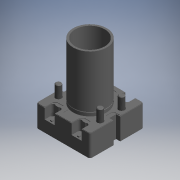
# Autodesk Inventor part: SLZ_63_Abdeckkappe#
Saved by Autodesk Inventor 2017.3 (Build 213256000, 256)
## iProperties
Part Number: SLZ_63_Abdeckkappe#
Material: Generic
Catalog Web Link: www.cadenas.de
Description: AbdeckKappe_SLZ63-Control-Tec
Vendor: ROSEKRIEGER
Document SubType Name: Modeling
Designer: partserver
Manufacturer: ROSEKRIEGER
Mass: 177.566 g
Surface Area: 701.344 cm^2
Volume: 177.566 cm^3
Density: 1 g/cm^3
Appearance: PSOLRGB-128-128-128
Category: PARTsolutions
Company: ROSEKRIEGER
Title: SLZ_63_Abdeckkappe#
Author: Cadenas PARTsolutions
Comments: Control-Tec
PSOL_IDENT_0: {$CADENAS_DATA\23d-libs\rose_krieger\linearkomponenten\pool_lineartechnik\_hubsaeule_zyliinder\elekt
PSOL_IDENT_1: rozylinder\elekzyl_slz63\parts\slz63_plfl_abdeck_kappe.prj},189 {VTYP=3D},{NB=SLZ_63_Abdeckkappe#},{
PSOL_IDENT_2: LINA=SLZ_63_Abdeckkappe#},{NN=AbdeckKappe_SLZ63},{DATE=02.12.2020 11:16:21},{GEOMDATE=06.03.2017 15:
PSOL_IDENT_3: 22:00},{VERSION=},{LINEID=10},{WBVAR=},{WBNUMERIC=}  {NB=SLZ_63_Abdeckkappe#},{LINA=SLZ_63_Abdeckkap
PSOL_IDENT_4: pe#},{KT=DUMMY},{IDNR=},{CODE=TQ3},{ARTIKEL=Elektrozylinder },{TYPE=SLZ 63 KG P PL},{BEST=SLZ_63_Abd
PSOL_IDENT_5: eckkappe},{VARIANTE=PL},{SPINDEL=KG 25x10},{SPINDELCODE=3.000},{SCHUTZARTVIS=IP54},{SCHUTZART=1},{HU
PSOL_IDENT_6: B1=0,[0:100]},{HINWEINBAUX=Hub + 288,5 mm},{DUMMYDURCH=10.000},{DUMMYLAENG=20.000},{HILFEHUB=105},{L
PSOL_IDENT_7: AENDOPPROFIL=184.500},{RF=1.000},{GRUNDKOE=288.500},{A=100},{B=80},{C=100},{D=125},{E=238},{F=40},{G=
PSOL_IDENT_8: M16x1.5},{H=104},{K=125},{L=105},{M=48},{N=56.5},{O=86},{P=18.5},{PPATH=sbl_lz70p_plfl.prj}
NB: SLZ_63_Abdeckkappe#
NN: AbdeckKappe_SLZ63
NT: Control-Tec
NBSYN: $BEST.#
LINA: SLZ_63_Abdeckkappe#
CATALOG: RK Rose+Krieger
ARTIKEL: Elektrozylinder
TYPE: SLZ 63 KG P PL
BEST: SLZ_63_Abdeckkappe
VARIANTE: PL
SPINDEL: KG 25x10
SPINDELCODE: 3
SCHUTZARTVIS: IP54
SCHUTZART: 1
HUB1: 0,[0:100]
HINWEINBAUX: Hub + 288,5 mm
DUMMYDURCH: 10
DUMMYLAENG: 20
HILFEHUB: 105
LAENDOPPROFIL: 184.5
RF: 1
GRUNDKOE: 288.5
A: 100
B: 80
C: 100
D: 125
E: 238
F: 40
G: M16x1.5
H: 104
K: 125
L: 105
M: 48
N: 56.5
O: 86
P: 18.5
SUPPLIER: ROSEKRIEGER
ARTICLENO: SLZ_63_Abdeckkappe#
BOMINFO: SLZ_63_Abdeckkappe#
CREATOR: CADENAS GmbH
Autodesk Inventor part; units mm, degrees
sketch "Sketch_2" plane through (0, 0, 0) normal (0, 0, 1) x (1, 0, 0)
  arc A0 (-40, -37) -> (-37, -40) centre (-37, -37) ccw
  line L0 (-37, -40) -> (37, -40)
  arc A1 (37, -40) -> (40, -37) centre (37, -37) ccw
  line L1 (40, -37) -> (40, -5)
  line L2 (40, -5) -> (33.9, -5)
  line L3 (33.9, -5) -> (33.9, 5)
  line L4 (33.9, 5) -> (40, 5)
  line L5 (40, 5) -> (40, 37)
  arc A2 (40, 37) -> (37, 40) centre (37, 37) ccw
  line L6 (37, 40) -> (-37, 40)
  arc A3 (-37, 40) -> (-40, 37) centre (-37, 37) ccw
  line L7 (-40, 37) -> (-40, 5)
  line L8 (-40, 5) -> (-33.9, 5)
  line L9 (-33.9, 5) -> (-33.9, -5)
  line L10 (-33.9, -5) -> (-40, -5)
  line L11 (-40, -5) -> (-40, -37)
  circle A4 centre (31, 16) radius 4.5
  circle A5 centre (31, -16) radius 4.5
  circle A6 centre (-31, 16) radius 4.5
  circle A7 centre (-31, -16) radius 4.5
  constraints: 24 end point, 8 centre point, 8 point on circle
extrude "Extrusion1" add sketch "Sketch_2" along normal blind 22
sketch "Sketch_1" plane through (0, 0, 22) normal (0, 0, 1) x (1, 0, 0)
  arc A0 (-40, -37) -> (-37, -40) centre (-37, -37) ccw
  line L0 (-37, -40) -> (37, -40)
  arc A1 (37, -40) -> (40, -37) centre (37, -37) ccw
  line L1 (40, -37) -> (40, -5)
  line L2 (40, -5) -> (33.9, -5)
  line L3 (33.9, -5) -> (33.9, 5)
  line L4 (33.9, 5) -> (40, 5)
  line L5 (40, 5) -> (40, 37)
  arc A2 (40, 37) -> (37, 40) centre (37, 37) ccw
  line L6 (37, 40) -> (-37, 40)
  arc A3 (-37, 40) -> (-40, 37) centre (-37, 37) ccw
  line L7 (-40, 37) -> (-40, 5)
  line L8 (-40, 5) -> (-33.9, 5)
  line L9 (-33.9, 5) -> (-33.9, -5)
  line L10 (-33.9, -5) -> (-40, -5)
  line L11 (-40, -5) -> (-40, -37)
  circle A4 centre (31, 16) radius 7.5
  circle A5 centre (31, -16) radius 7.5
  circle A6 centre (-31, 16) radius 7.5
  circle A7 centre (-31, -16) radius 7.5
  constraints: 24 end point, 8 centre point, 8 point on circle
extrude "Extrusion2" add sketch "Sketch_1" along normal blind 10
sketch "Sketch_3" plane through (0, 0, 0) normal (1, 0, 0) x (0, 0, -1)
  line L0 (6, 0) -> (-47, 0)
  line L1 (-47, 0) -> (-47, 22.5)
  line L2 (-47, 22.5) -> (-32.5, 22.5)
  arc A0 (-32.5, 22.5) -> (-32, 23) centre (-32.5, 23) ccw
  line L3 (-32, 23) -> (-32, 27)
  line L4 (-32, 27) -> (0, 27)
  line L5 (0, 27) -> (0, 25.1)
  arc A1 (0, 25.1) -> (0.3, 24.8) centre (0.3, 25.1) ccw
  line L6 (0.3, 24.8) -> (5, 24.8)
  line L7 (5, 24.8) -> (6, 23.8)
  line L8 (6, 23.8) -> (6, 0)
  line L9 (6, 0) -> (-47, 0)
  constraints: 20 end point, 4 point on circle, 2 centre point
revolve "Revolution1" add sketch "Sketch_3" angle 360 about axis through (0, 0, -6) along (0, 0, -1)
sketch "Sketch_4" plane through (0, 0, 0) normal (1, 0, 0) x (0, 0, -1)
  line L0 (6, 0) -> (-47, 0)
  line L1 (-47, 0) -> (-47, 21.7871)
  line L2 (-47, 21.7871) -> (-44.7, 20.95)
  line L3 (-44.7, 20.95) -> (-44.5, 20.95)
  line L4 (-44.5, 20.95) -> (-44.5, 22)
  line L5 (-44.5, 22) -> (-43, 22)
  line L6 (-43, 22) -> (-43, 20.75)
  line L7 (-43, 20.75) -> (-41.2, 20.75)
  line L8 (-41.2, 20.75) -> (-41, 20.95)
  line L9 (-41, 20.95) -> (-41, 21.5)
  line L10 (-41, 21.5) -> (-33, 21.5)
  line L11 (-33, 21.5) -> (-33, 20.95)
  line L12 (-33, 20.95) -> (-32.8, 20.75)
  line L13 (-32.8, 20.75) -> (-30.2, 20.75)
  line L14 (-30.2, 20.75) -> (-30, 20.95)
  line L15 (-30, 20.95) -> (-30, 22)
  line L16 (-30, 22) -> (-8.2, 22)
  line L17 (-8.2, 22) -> (-8, 22.2)
  line L18 (-8, 22.2) -> (-8, 24.95)
  arc A0 (-7.7, 25.25) -> (-8, 24.95) centre (-7.7, 24.95) ccw
  line L19 (-7.7, 25.25) -> (-2.3, 25.25)
  arc A1 (-2, 24.95) -> (-2.3, 25.25) centre (-2.3, 24.95) ccw
  line L20 (-2, 24.95) -> (-2, 22.2)
  line L21 (-2, 22.2) -> (-1.8, 22)
  line L22 (-1.8, 22) -> (6, 22)
  line L23 (6, 22) -> (6, 0)
  line L24 (6, 0) -> (-47, 0)
  constraints: 50 end point, 4 point on circle, 2 centre point
revolve "Revolution2" cut sketch "Sketch_4" angle 360 about axis through (0, 0, -6) along (0, 0, -1)
sketch "Sketch_5" plane through (0, 0, 0) normal (0, 0, 1) x (1, 0, 0)
  line L0 (-50, -50) -> (50, -50)
  line L1 (50, -50) -> (50, 50)
  line L2 (50, 50) -> (-50, 50)
  line L3 (-50, 50) -> (-50, -50)
  line L4 (-40, 40) -> (-40, -40)
  line L5 (-40, -40) -> (-27.5, -40)
  line L6 (-27.5, -40) -> (-27.5, -31)
  arc A0 (-22.2639, -29) -> (-27.5, -31) centre (-24.5, -31) ccw
  line L7 (-22.2639, -29) -> (-17.7361, -29)
  arc A1 (-12.5, -31) -> (-17.7361, -29) centre (-15.5, -31) ccw
  line L8 (-12.5, -31) -> (-12.5, -40)
  line L9 (-12.5, -40) -> (12.5, -40)
  line L10 (12.5, -40) -> (12.5, -31)
  arc A2 (17.7361, -29) -> (12.5, -31) centre (15.5, -31) ccw
  line L11 (17.7361, -29) -> (22.2639, -29)
  arc A3 (27.5, -31) -> (22.2639, -29) centre (24.5, -31) ccw
  line L12 (27.5, -31) -> (27.5, -40)
  line L13 (27.5, -40) -> (40, -40)
  line L14 (40, -40) -> (40, 40)
  line L15 (40, 40) -> (27.5, 40)
  line L16 (27.5, 40) -> (27.5, 31)
  arc A4 (22.2639, 29) -> (27.5, 31) centre (24.5, 31) ccw
  line L17 (22.2639, 29) -> (17.7361, 29)
  arc A5 (12.5, 31) -> (17.7361, 29) centre (15.5, 31) ccw
  line L18 (12.5, 31) -> (12.5, 40)
  line L19 (12.5, 40) -> (-12.5, 40)
  line L20 (-12.5, 40) -> (-12.5, 31)
  arc A6 (-17.7361, 29) -> (-12.5, 31) centre (-15.5, 31) ccw
  line L21 (-17.7361, 29) -> (-22.2639, 29)
  arc A7 (-27.5, 31) -> (-22.2639, 29) centre (-24.5, 31) ccw
  line L22 (-27.5, 31) -> (-27.5, 40)
  line L23 (-27.5, 40) -> (-40, 40)
  constraints: 48 end point, 16 point on circle, 8 centre point
extrude "Extrusion3" cut sketch "Sketch_5" along normal blind 13.5
sketch "Sketch_6" plane through (0, 0, 13.5) normal (0, 0, 1) x (1, 0, 0)
  line L0 (-50, -50) -> (50, -50)
  line L1 (50, -50) -> (50, 50)
  line L2 (50, 50) -> (-50, 50)
  line L3 (-50, 50) -> (-50, -50)
  line L4 (18.5, 35.5) -> (21.5, 35.5)
  line L5 (21.5, 35.5) -> (21.5, 38)
  line L6 (21.5, 38) -> (18.5, 38)
  line L7 (18.5, 38) -> (18.5, 35.5)
  line L8 (18.5, -35.5) -> (18.5, -38)
  line L9 (18.5, -38) -> (21.5, -38)
  line L10 (21.5, -38) -> (21.5, -35.5)
  line L11 (21.5, -35.5) -> (18.5, -35.5)
  line L12 (-21.5, 35.5) -> (-18.5, 35.5)
  line L13 (-18.5, 35.5) -> (-18.5, 38)
  line L14 (-18.5, 38) -> (-21.5, 38)
  line L15 (-21.5, 38) -> (-21.5, 35.5)
  line L16 (-21.5, -35.5) -> (-21.5, -38)
  line L17 (-21.5, -38) -> (-18.5, -38)
  line L18 (-18.5, -38) -> (-18.5, -35.5)
  line L19 (-18.5, -35.5) -> (-21.5, -35.5)
  line L20 (-40, 40) -> (-40, -40)
  line L21 (-40, -40) -> (-27.5, -40)
  line L22 (-27.5, -40) -> (-27.5, -31)
  arc A0 (-22.2639, -29) -> (-27.5, -31) centre (-24.5, -31) ccw
  line L23 (-22.2639, -29) -> (-17.7361, -29)
  arc A1 (-12.5, -31) -> (-17.7361, -29) centre (-15.5, -31) ccw
  line L24 (-12.5, -31) -> (-12.5, -40)
  line L25 (-12.5, -40) -> (12.5, -40)
  line L26 (12.5, -40) -> (12.5, -31)
  arc A2 (17.7361, -29) -> (12.5, -31) centre (15.5, -31) ccw
  line L27 (17.7361, -29) -> (22.2639, -29)
  arc A3 (27.5, -31) -> (22.2639, -29) centre (24.5, -31) ccw
  line L28 (27.5, -31) -> (27.5, -40)
  line L29 (27.5, -40) -> (40, -40)
  line L30 (40, -40) -> (40, 40)
  line L31 (40, 40) -> (27.5, 40)
  line L32 (27.5, 40) -> (27.5, 31)
  arc A4 (22.2639, 29) -> (27.5, 31) centre (24.5, 31) ccw
  line L33 (22.2639, 29) -> (17.7361, 29)
  arc A5 (12.5, 31) -> (17.7361, 29) centre (15.5, 31) ccw
  line L34 (12.5, 31) -> (12.5, 40)
  line L35 (12.5, 40) -> (-12.5, 40)
  line L36 (-12.5, 40) -> (-12.5, 31)
  arc A6 (-17.7361, 29) -> (-12.5, 31) centre (-15.5, 31) ccw
  line L37 (-17.7361, 29) -> (-22.2639, 29)
  arc A7 (-27.5, 31) -> (-22.2639, 29) centre (-24.5, 31) ccw
  line L38 (-27.5, 31) -> (-27.5, 40)
  line L39 (-27.5, 40) -> (-40, 40)
  constraints: 80 end point, 16 point on circle, 8 centre point
extrude "Extrusion4" cut sketch "Sketch_6" along normal blind 1.5
sketch "Sketch7" plane through (0, 0, 32) normal (0, 0, 1) x (1, 0, 0)
  point P0 (28.25, 28.25)
hole "Hole1" at (28.25, 28.25, 32) direction (0, 0, -1) diameter 6.8 depth 20 tip angle 118
pattern_linear "Rectangular Pattern1" count 2 spacing 56.5 along (-1, 0, 0) count 2 spacing 56.5 along (0, -1, 0) of "Hole1"
sketch "Sketch_7" plane through (0, 0, 0) normal (0, 0, 1) x (1, 0, 0)
  arc A0 (-39.6, -36.6) -> (-36.6, -39.6) centre (-36.6, -36.6) ccw
  line L0 (-36.6, -39.6) -> (-31, -39.6)
  arc A1 (-31, -39.6) -> (-28, -36.6) centre (-31, -36.6) ccw
  line L1 (-28, -36.6) -> (-28, -28.8426)
  arc A2 (-27.1213, -26.7213) -> (-28, -28.8426) centre (-25, -28.8426) ccw
  line L2 (-27.1213, -26.7213) -> (-24.6929, -24.2929)
  arc A3 (-23.9858, -24) -> (-24.6929, -24.2929) centre (-23.9858, -25) ccw
  line L3 (-23.9858, -24) -> (-16.0142, -24)
  arc A4 (-15.3071, -24.2929) -> (-16.0142, -24) centre (-16.0142, -25) ccw
  line L4 (-15.3071, -24.2929) -> (-12.8787, -26.7213)
  arc A5 (-12, -28.8426) -> (-12.8787, -26.7213) centre (-15, -28.8426) ccw
  line L5 (-12, -28.8426) -> (-12, -36.6)
  arc A6 (-12, -36.6) -> (-9, -39.6) centre (-9, -36.6) ccw
  line L6 (-9, -39.6) -> (9, -39.6)
  arc A7 (9, -39.6) -> (12, -36.6) centre (9, -36.6) ccw
  line L7 (12, -36.6) -> (12, -28.8426)
  arc A8 (12.8787, -26.7213) -> (12, -28.8426) centre (15, -28.8426) ccw
  line L8 (12.8787, -26.7213) -> (15.3071, -24.2929)
  arc A9 (16.0142, -24) -> (15.3071, -24.2929) centre (16.0142, -25) ccw
  line L9 (16.0142, -24) -> (23.9858, -24)
  arc A10 (24.6929, -24.2929) -> (23.9858, -24) centre (23.9858, -25) ccw
  line L10 (24.6929, -24.2929) -> (27.1213, -26.7213)
  arc A11 (28, -28.8426) -> (27.1213, -26.7213) centre (25, -28.8426) ccw
  line L11 (28, -28.8426) -> (28, -36.6)
  arc A12 (28, -36.6) -> (31, -39.6) centre (31, -36.6) ccw
  line L12 (31, -39.6) -> (36.6, -39.6)
  arc A13 (36.6, -39.6) -> (39.6, -36.6) centre (36.6, -36.6) ccw
  line L13 (39.6, -36.6) -> (39.6, -9.1)
  arc A14 (39.6, -9.1) -> (36.6, -6.1) centre (36.6, -9.1) ccw
  line L14 (36.6, -6.1) -> (31.6, -6.1)
  arc A15 (28.6, -3.1) -> (31.6, -6.1) centre (31.6, -3.1) ccw
  line L15 (28.6, -3.1) -> (28.6, 3.1)
  arc A16 (31.6, 6.1) -> (28.6, 3.1) centre (31.6, 3.1) ccw
  line L16 (31.6, 6.1) -> (36.6, 6.1)
  arc A17 (36.6, 6.1) -> (39.6, 9.1) centre (36.6, 9.1) ccw
  line L17 (39.6, 9.1) -> (39.6, 36.6)
  arc A18 (39.6, 36.6) -> (36.6, 39.6) centre (36.6, 36.6) ccw
  line L18 (36.6, 39.6) -> (31, 39.6)
  arc A19 (31, 39.6) -> (28, 36.6) centre (31, 36.6) ccw
  line L19 (28, 36.6) -> (28, 28.8426)
  arc A20 (27.1213, 26.7213) -> (28, 28.8426) centre (25, 28.8426) ccw
  line L20 (27.1213, 26.7213) -> (24.6929, 24.2929)
  arc A21 (23.9858, 24) -> (24.6929, 24.2929) centre (23.9858, 25) ccw
  line L21 (23.9858, 24) -> (16.0142, 24)
  arc A22 (15.3071, 24.2929) -> (16.0142, 24) centre (16.0142, 25) ccw
  line L22 (15.3071, 24.2929) -> (12.8787, 26.7213)
  arc A23 (12, 28.8426) -> (12.8787, 26.7213) centre (15, 28.8426) ccw
  line L23 (12, 28.8426) -> (12, 36.6)
  arc A24 (12, 36.6) -> (9, 39.6) centre (9, 36.6) ccw
  line L24 (9, 39.6) -> (-9, 39.6)
  arc A25 (-9, 39.6) -> (-12, 36.6) centre (-9, 36.6) ccw
  line L25 (-12, 36.6) -> (-12, 28.8426)
  arc A26 (-12.8787, 26.7213) -> (-12, 28.8426) centre (-15, 28.8426) ccw
  line L26 (-12.8787, 26.7213) -> (-15.3071, 24.2929)
  arc A27 (-16.0142, 24) -> (-15.3071, 24.2929) centre (-16.0142, 25) ccw
  line L27 (-16.0142, 24) -> (-23.9858, 24)
  arc A28 (-24.6929, 24.2929) -> (-23.9858, 24) centre (-23.9858, 25) ccw
  line L28 (-24.6929, 24.2929) -> (-27.1213, 26.7213)
  arc A29 (-28, 28.8426) -> (-27.1213, 26.7213) centre (-25, 28.8426) ccw
  line L29 (-28, 28.8426) -> (-28, 36.6)
  arc A30 (-28, 36.6) -> (-31, 39.6) centre (-31, 36.6) ccw
  line L30 (-31, 39.6) -> (-36.6, 39.6)
  arc A31 (-36.6, 39.6) -> (-39.6, 36.6) centre (-36.6, 36.6) ccw
  line L31 (-39.6, 36.6) -> (-39.6, 9.1)
  arc A32 (-39.6, 9.1) -> (-36.6, 6.1) centre (-36.6, 9.1) ccw
  line L32 (-36.6, 6.1) -> (-31.6, 6.1)
  arc A33 (-28.6, 3.1) -> (-31.6, 6.1) centre (-31.6, 3.1) ccw
  line L33 (-28.6, 3.1) -> (-28.6, -3.1)
  arc A34 (-31.6, -6.1) -> (-28.6, -3.1) centre (-31.6, -3.1) ccw
  line L34 (-31.6, -6.1) -> (-36.6, -6.1)
  arc A35 (-36.6, -6.1) -> (-39.6, -9.1) centre (-36.6, -9.1) ccw
  line L35 (-39.6, -9.1) -> (-39.6, -36.6)
  circle A36 centre (31, -16) radius 4.5
  circle A37 centre (31, 16) radius 4.5
  arc A38 (-9.2062, 23.5119) -> (-9.2062, -23.5119) centre (0, 0) ccw
  arc A39 (-7.3, -26.3054) -> (-9.2062, -23.5119) centre (-10.3, -26.3054) ccw
  line L36 (-7.3, -26.3054) -> (-7.3, -30.5)
  arc A40 (-7.3, -30.5) -> (-4.3, -33.5) centre (-4.3, -30.5) ccw
  line L37 (-4.3, -33.5) -> (4.3, -33.5)
  arc A41 (4.3, -33.5) -> (7.3, -30.5) centre (4.3, -30.5) ccw
  line L38 (7.3, -30.5) -> (7.3, -26.3054)
  arc A42 (9.2062, -23.5119) -> (7.3, -26.3054) centre (10.3, -26.3054) ccw
  arc A43 (9.2062, -23.5119) -> (9.2062, 23.5119) centre (0, 0) ccw
  arc A44 (7.3, 26.3054) -> (9.2062, 23.5119) centre (10.3, 26.3054) ccw
  line L39 (7.3, 26.3054) -> (7.3, 30.5)
  arc A45 (7.3, 30.5) -> (4.3, 33.5) centre (4.3, 30.5) ccw
  line L40 (4.3, 33.5) -> (-4.3, 33.5)
  arc A46 (-4.3, 33.5) -> (-7.3, 30.5) centre (-4.3, 30.5) ccw
  line L41 (-7.3, 30.5) -> (-7.3, 26.3054)
  arc A47 (-9.2062, 23.5119) -> (-7.3, 26.3054) centre (-10.3, 26.3054) ccw
  circle A48 centre (-31, 16) radius 4.5
  circle A49 centre (-31, -16) radius 4.5
  constraints: 92 point on circle, 84 end point, 50 centre point
extrude "Extrusion5" add sketch "Sketch_7" against normal blind 0.5
sketch "Sketch_10" plane through (0, 0, 0) normal (1, 0, 0) x (0, 0, -1)
  line L0 (-43, 0) -> (-50.5, 0)
  line L1 (-50.5, 19.9) -> (-46.9931, 20.3991)
  line L2 (-46.9931, 20.3991) -> (-43, 19.9)
  line L3 (-43, 19.9) -> (-43, 21.95)
  line L4 (-43, 21.95) -> (-44.5, 21.95)
  line L5 (-44.5, 21.95) -> (-44.5, 21.4685)
  arc A0 (-44.9026, 21.1866) -> (-44.5, 21.4685) centre (-44.8, 21.4685) ccw
  line L6 (-44.9026, 21.1866) -> (-47, 21.95)
  line L7 (-47, 21.95) -> (-47, 22.5)
  line L8 (-47, 22.5) -> (-47.476, 22.5)
  arc A1 (-47.476, 22.5) -> (-48.7438, 22.2189) centre (-47.476, 19.5) ccw
  line L9 (-48.7438, 22.2189) -> (-49.9226, 21.6692)
  arc A2 (-49.9226, 21.6692) -> (-50.5, 20.7629) centre (-49.5, 20.7629) ccw
  line L10 (-50.5, 20.7629) -> (-50.5, 19.9)
  constraints: 22 end point, 6 point on circle, 3 centre point
revolve "Revolution3" add sketch "Sketch_10" angle 360 about axis through (0, 0, 43) along (0, 0, -1)
sketch "Sketch_11" plane through (0, 0, 0) normal (1, 0, 0) x (0, 0, -1)
  line L0 (84, 0) -> (6, 0)
  line L1 (6, 22) -> (84, 22)
  line L2 (84, 22) -> (84, 25)
  line L3 (84, 25) -> (6, 25)
  line L4 (6, 25) -> (6, 22)
  constraints: 10 end point
revolve "Revolution4" add sketch "Sketch_11" angle 360 about axis through (0, 0, -84) along (0, 0, -1)
sketch "Sketch_13" plane through (31, 0, 0) normal (1, 0, 0) x (0, 0, -1)
  line L0 (18, 16) -> (-30, 16)
  line L1 (-30, 16) -> (-30, 21.7)
  line L2 (-30, 21.7) -> (-29.2, 22.5)
  line L3 (-29.2, 22.5) -> (-22.4, 22.5)
  arc A0 (-22, 22.1) -> (-22.4, 22.5) centre (-22.4, 22.1) ccw
  line L4 (-22, 22.1) -> (-22, 20.4)
  arc A1 (-22, 20.4) -> (-21.6, 20) centre (-21.6, 20.4) ccw
  line L5 (-21.6, 20) -> (17.233, 20)
  line L6 (17.233, 20) -> (18, 19.233)
  line L7 (18, 19.233) -> (18, 16)
  line L8 (18, 16) -> (-30, 16)
  constraints: 18 end point, 4 point on circle, 2 centre point
revolve "Revolution5" add sketch "Sketch_13" angle 360 about axis through (31, 16, -18) along (0, 0, -1)
thread "Thread1" size "M8x1.25" class "6g" standard "ISO Metric profile" length 38.6716 offset 0.9284
pattern_linear "Rectangular Pattern2" count 2 spacing 62 along (-1, 0, 0) count 2 spacing 32 along (0, -1, 0) of "Revolution5"
sketch "Sketch_17" plane through (0, 0, 30) normal (0, 0, 1) x (1, 0, 0)
  line L0 (28, 14.2679) -> (31, 12.5359)
  line L1 (31, 12.5359) -> (34, 14.2679)
  line L2 (34, 14.2679) -> (34, 17.7321)
  line L3 (34, 17.7321) -> (31, 19.4641)
  line L4 (31, 19.4641) -> (28, 17.7321)
  line L5 (28, 17.7321) -> (28, 14.2679)
  constraints: 12 end point
extrude "Extrusion6" cut sketch "Sketch_17" against normal blind 4
pattern_linear "Rectangular Pattern3" count 2 spacing 62 along (-1, 0, 0) count 2 spacing 32 along (0, -1, 0) of "Extrusion6"
ref_plane "ABDECKSTOEPSEL1_XY" through (-20, 40, 0) normal (0, 0, 1) x (1, 0, 0)
ref_plane "ABDECKSTOEPSEL1_YZ" through (-20, 40, 0) normal (1, 0, 0) x (0, 1, 0)
ref_plane "ABDECKSTOEPSEL1_ZX" through (-20, 40, 0) normal (0, 1, 0) x (0, 0, 1)
ref_plane "ABDECKSTOEPSEL2_XY" through (20, 40, 0) normal (0, 0, 1) x (1, 0, 0)
ref_plane "ABDECKSTOEPSEL2_YZ" through (20, 40, 0) normal (1, 0, 0) x (0, 1, 0)
ref_plane "ABDECKSTOEPSEL2_ZX" through (20, 40, 0) normal (0, 1, 0) x (0, 0, 1)
ref_plane "ABDECKSTOEPSEL3_XY" through (20, -40, 0) normal (0, 0, 1) x (1, 0, 0)
ref_plane "ABDECKSTOEPSEL3_YZ" through (20, -40, 0) normal (1, 0, 0) x (0, 1, 0)
ref_plane "ABDECKSTOEPSEL3_ZX" through (20, -40, 0) normal (0, 1, 0) x (0, 0, 1)
ref_plane "ABDECKSTOEPSEL4_XY" through (-20, -40, 0) normal (0, 0, 1) x (1, 0, 0)
ref_plane "ABDECKSTOEPSEL4_YZ" through (-20, -40, 0) normal (1, 0, 0) x (0, 1, 0)
ref_plane "ABDECKSTOEPSEL4_ZX" through (-20, -40, 0) normal (0, 1, 0) x (0, 0, 1)
ref_plane "BP_POSHUB_MA_XY" through (0, 0, 32) normal (0, 0, -1) x (1, 0, 0)
ref_plane "BP_POSHUB_MA_YZ" through (0, 0, 32) normal (1, 0, 0) x (0, -1, 0)
ref_plane "BP_POSHUB_MA_ZX" through (0, 0, 32) normal (0, -1, 0) x (0, 0, -1)
ref_plane "DP451_5_XY" through (-22.5, 0, 40) normal (0, 1, 0) x (1, 0, 0)
ref_plane "DP451_5_YZ" through (-22.5, 0, 40) normal (1, 0, 0) x (0, 0, -1)
ref_plane "DP451_5_ZX" through (-22.5, 0, 40) normal (0, 0, -1) x (0, 1, 0)
ref_plane "DP452_5_XY" through (22.5, 0, 40) normal (0, 1, 0) x (1, 0, 0)
ref_plane "DP452_5_YZ" through (22.5, 0, 40) normal (1, 0, 0) x (0, 0, -1)
ref_plane "DP452_5_ZX" through (22.5, 0, 40) normal (0, 0, -1) x (0, 1, 0)
ref_plane "DPM1_XY" through (0, 40, 32) normal (1, 0, 0) x (0, 0, -1)
ref_plane "DPM1_YZ" through (0, 40, 32) normal (0, 0, -1) x (0, 1, 0)
ref_plane "DPM1_ZX" through (0, 40, 32) normal (0, 1, 0) x (1, 0, 0)
ref_plane "DPNULL2_XY" through (0, -20, 50.5) normal (1, 0, 0) x (0, 0, -1)
ref_plane "DPNULL2_YZ" through (0, -20, 50.5) normal (0, 0, -1) x (0, 1, 0)
ref_plane "DPNULL2_ZX" through (0, -20, 50.5) normal (0, 1, 0) x (1, 0, 0)
ref_plane "DPP1_XY" through (0, 40, 32) normal (1, 0, 0) x (0, 0, -1)
ref_plane "DPP1_YZ" through (0, 40, 32) normal (0, 0, -1) x (0, 1, 0)
ref_plane "DPP1_ZX" through (0, 40, 32) normal (0, 1, 0) x (1, 0, 0)
ref_plane "DPP2_XY" through (0, 20, 50.5) normal (1, 0, 0) x (0, 0, -1)
ref_plane "DPP2_YZ" through (0, 20, 50.5) normal (0, 0, -1) x (0, 1, 0)
ref_plane "DPP2_ZX" through (0, 20, 50.5) normal (0, 1, 0) x (1, 0, 0)
ref_plane "PROFIL_XY" through (0, 0, -0.5) normal (0, 0, 1) x (1, 0, 0)
ref_plane "PROFIL_YZ" through (0, 0, -0.5) normal (1, 0, 0) x (0, 1, 0)
ref_plane "PROFIL_ZX" through (0, 0, -0.5) normal (0, 1, 0) x (0, 0, 1)
ref_plane "SCHUBSTANGE_XY" through (0, 0, 47) normal (0, 0, -1) x (1, 0, 0)
ref_plane "SCHUBSTANGE_YZ" through (0, 0, 47) normal (1, 0, 0) x (0, -1, 0)
ref_plane "SCHUBSTANGE_ZX" through (0, 0, 47) normal (0, -1, 0) x (0, 0, -1)
body "Solid1"
